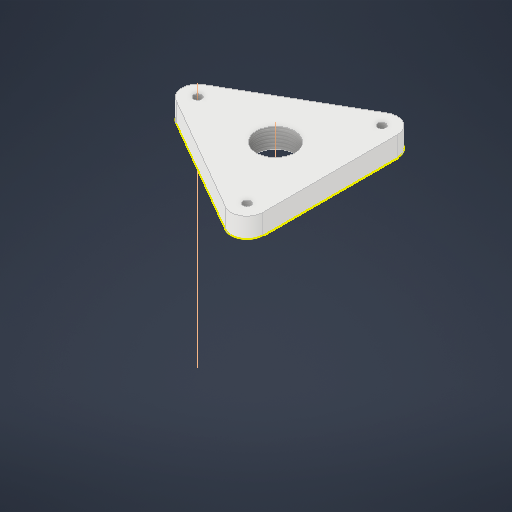
# Autodesk Inventor part: Triangle_RK
Saved by Autodesk Inventor 2026 (Build 300175050, 175E)
## iProperties
Created: 2019-01-09
Part Number: Triangle_RK
Material: white material
Document SubType Name: Modeling
Designer: Vi Quint Duong
Density: 1 g/cm^3
Appearance: Generic
Author: Vi Quint Duong
Autodesk Inventor part; units mm, degrees
ref_plane "YZ Plane" through (0, 0, 0) normal (1, 0, 0) x (0, 1, 0)
ref_plane "XZ Plane" through (0, 0, 0) normal (0, 1, 0) x (-1, 0, 0)
sketch "Sketch1" plane through (0, 0, 0) normal (0, 1, 0) x (-1, 0, 0)
  circle A0 centre (1.4663, 0.135) radius 40 projected
  circle A1 centre (1.4663, 0.135) radius 60 projected
  line L0 (55.7483, -8.5253) -> (-18.1747, -51.2048)
  line L1 (-33.1747, -42.5445) -> (-33.1747, 42.8145)
  line L2 (-18.1747, 51.4747) -> (55.7483, 8.7952)
  arc A2 (55.7483, -8.5253) -> (55.7483, 8.7952) centre (50.7483, 0.135) ccw
  arc A3 (-33.1747, -42.5445) -> (-18.1747, -51.2048) centre (-23.1747, -42.5445) ccw
  arc A4 (-18.1747, 51.4747) -> (-33.1747, 42.8145) centre (-23.1747, 42.8145) ccw
  point P0 (70.7483, 0.135)
  point P1 (-33.1747, -59.865)
  point P2 (-33.1747, 60.135)
  dimension "d2" = 120
  dimension "d3" = 10
  constraints: 6 end point, 6 point on circle, 6 point on line, 6 tangent, 3 centre point, 2 equal radius, 1 coincident, 7 other
  measures "d2" distance of point (-33.175, -59.865) point (-33.175, 60.135)
  measures "d3" radius of A2
extrude "Extrusion1" add sketch "Sketch1" along normal blind 12.7 contours A0 L0 L1 L2 | A0 L2 A2 L0 | A0 L1 A4 L2 | L0 A3 L1 A0
sketch "Sketch4" plane through (0, 0, 0) normal (0, -1, 0) x (1, 0, 0)
  line L0 (-55.7483, -8.5253) -> (18.1747, -51.2048) projected
  arc A0 (18.1747, -51.2048) -> (33.1747, -42.5445) centre (23.1747, -42.5445) ccw projected
  line L1 (33.1747, -42.5445) -> (33.1747, 42.8145) projected
  arc A1 (33.1747, 42.8145) -> (18.1747, 51.4747) centre (23.1747, 42.8145) ccw projected
  line L2 (18.1747, 51.4747) -> (-55.7483, 8.7952) projected
  arc A2 (-55.7483, 8.7952) -> (-55.7483, -8.5253) centre (-50.7483, 0.135) ccw projected
  point P0 (0, 0)
ref_plane "Work Plane1" through (-50.7483, 0, 0.135) normal (1, 0, 0) x (0, 0, -1)
sketch "Sketch6" plane through (0, 12.7, 0) normal (0, 1, 0) x (1, 0, 0)
  line L0 (18.1747, 51.2048) -> (-55.7483, 8.5253) projected
  arc A0 (-55.7483, 8.5253) -> (-55.7483, -8.7952) centre (-50.7483, -0.135) ccw projected
  line L1 (-55.7483, -8.7952) -> (18.1747, -51.4747) projected
  arc A1 (18.1747, -51.4747) -> (33.1747, -42.8145) centre (23.1747, -42.8145) ccw projected
  line L2 (33.1747, -42.8145) -> (33.1747, 42.5445) projected
  arc A2 (33.1747, 42.5445) -> (18.1747, 51.2048) centre (23.1747, 42.5445) ccw projected
  line L3 (23.1747, 42.5445) -> (23.1747, -42.8145) construction
  circle A3 centre (-50.7483, -0.135) radius 1.5 construction
  line L4 (-50.7483, -0.135) -> (23.1747, -0.135) construction
  line L5 (23.1747, 42.5445) -> (-50.7483, -0.135) construction
  line L6 (23.1747, -42.8145) -> (-13.7868, 21.2048) construction
  line L7 (-50.7483, -0.135) -> (23.1747, -42.8145) construction
  line L8 (23.1747, 42.5445) -> (-13.7868, -21.4747) construction
  circle A4 centre (-1.4663, -0.135) radius 17.5
  point P0 (0, 0)
  dimension "d38" = 35
  constraints: 12 end point, 3 midpoint, 3 point on line, 1 centre point, 1 coincident, 1 vertical
  measures "d38" diameter of A4
hole "Hole1" at (-1.4663, 12.7, 0.135) direction (0, -1, 0) diameter 24.25 end through all
hole "Hole2" at (-50.7483, 12.7, 0.135) at (23.1747, 12.7, 42.8145) at (23.1747, 12.7, -42.5445) direction (0, -1, 0) diameter 5 end through all
thread "Thread1" size "M6x1" class "6H" standard "ANSI Metric M Profile" full length
thread "Thread2" size "M6x1" class "6H" standard "ANSI Metric M Profile" full length
thread "Thread3" size "M6x1" class "6H" standard "ANSI Metric M Profile" full length
thicken "Thicken1" operation add thickness 0.2 both sides no extend neighbours yes toward (0, -1, 0) faces at (25.6399, 12.7, 0.6222)
thread "Thread4" size "M25x2" class "6H" standard "ISO Metric profile" full length
body "Solid1"
